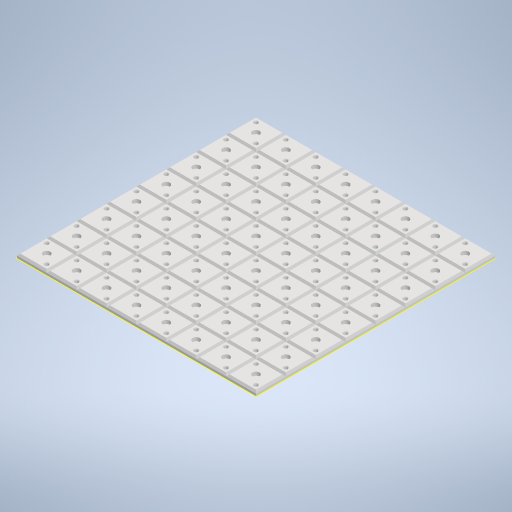
# Autodesk Inventor part: board-V2
Saved by Autodesk Inventor 2024.1 (Build 281209000, 209)
## iProperties
Created: 2025-07-31
Part Number: board-V2
Material: Generic
Document SubType Name: Modeling
Designer: iwheard
Density: 1 g/cm^3
Appearance: Default
Author: iwheard
Autodesk Inventor part; units mm, degrees
ref_plane "YZ Plane" through (0, 0, 0) normal (1, 0, 0) x (0, 1, 0)
ref_plane "XZ Plane" through (0, 0, 0) normal (0, 1, 0) x (-1, 0, 0)
ref_plane "XY Plane" through (0, 0, 0) normal (0, 0, 1) x (1, 0, 0)
sketch "Sketch1" plane through (0, 0, 0) normal (0, 1, 0) x (-1, 0, 0)
  line L0 (0, 0) -> (-25.5, 0)
  line L1 (-25.5, 0) -> (-25.5, -25.5)
  line L2 (-25.5, -25.5) -> (0, -25.5)
  line L3 (0, -25.5) -> (0, 0)
  dimension "d0" = 25.5
  dimension "d1" = 25.5
  constraints: 8 end point, 2 parallel, 1 horizontal, 1 perpendicular
  measures "d0" distance between parallel lines of L0 L2
  measures "d1" distance between parallel lines of L1 L3
extrude "Extrusion1" add sketch "Sketch1" along normal blind 3.5
chamfer "Chamfer1" distance 1.5 angle 45 4 edges at (12.75, 3.5, 0) (0, 3.5, -12.75) (25.5, 3.5, -12.75) (12.75, 3.5, -25.5)
sketch "Sketch2" plane through (0, 3.5, 0) normal (0, 1, 0) x (1, 0, 0)
  circle A0 centre (12.75, 12.75) radius 3
  line L0 (0, 0) -> (25.5, 0) projected
  line L1 (25.5, 25.5) -> (0, 25.5) projected
  line L2 (25.5, 0) -> (25.5, 25.5) projected
  line L3 (0, 25.5) -> (0, 0) projected
  dimension "d7" = 6
  dimension "d8" = 25.5
  dimension "d9" = 12.75
  dimension "d10" = 25.5
  dimension "d11" = 12.75
  constraints: 1 centre point
  measures "d7" diameter of A0
  measures "d8" distance between parallel lines of L0 L1
  measures "d9" distance from line of L1 A0.centre
  measures "d10" distance between parallel lines of L2 L3
  measures "d11" distance from line of L2 A0.centre
extrude "Extrusion2" cut sketch "Sketch2" against normal blind 3 contours A0
sketch "Sketch3" plane through (0, 3.5, 0) normal (0, 1, 0) x (1, 0, 0)
  circle A0 centre (20.5, 5) radius 1.5
  circle A1 centre (5, 20.5) radius 1.5
  line L0 (1.5, 24) -> (0, 25.5) projected
  line L1 (0, 25.5) -> (25.5, 0) construction
  line L2 (0, 0) -> (25.5, 0) projected
  dimension "d14" = 3
  dimension "d15" = 3
  dimension "d16" = 5
  dimension "d17" = 5
  constraints: 2 centre point, 2 end point, 2 point on line, 1 collinear
  measures "d14" diameter of A1
  measures "d15" diameter of A0
  measures "d16" horizontal distance of L0.end A1.centre
  measures "d17" distance from line of L2 A0.centre
extrude "Extrusion3" cut sketch "Sketch3" against normal blind 3
chamfer "Chamfer2" distance 0.5 angle 45 2 edges at (3.5, 3.5, -20.5) (19, 3.5, -5)
sketch "Sketch4" plane through (0, 0, 0) normal (0, -1, 0) x (1, 0, 0)
  line L0 (0, 0) -> (204, 0) projected
  line L1 (0, -204) -> (0, 0) projected
  line L2 (204, -204) -> (0, -204) projected
  line L3 (204, 0) -> (204, -204) projected
  line L4 (217, 13) -> (-13, 13)
  line L5 (-13, 13) -> (-13, -217)
  line L6 (-13, -217) -> (217, -217)
  line L7 (217, -217) -> (217, 13)
  dimension "d29" = 13
  constraints: 8 end point, 3 other
  measures "d29" distance between parallel lines of L4 L0
pattern_linear "Rectangular Pattern1" count 8 spacing 25.5 along (1, 0, 0) count 8 spacing 25.5 along (0, 0, -1)
sketch "Sketch5" plane through (0, 0, 0) normal (0, -1, 0) x (1, 0, 0)
  line L0 (0, 0) -> (204, 0) projected
  line L1 (0, -204) -> (0, 0) projected
  line L2 (204, -204) -> (0, -204) projected
  line L3 (204, 0) -> (204, -204) projected
equation "\"d9\" = 0.5 * d8"
equation "\"d11\" = 0.5 * d10"
body "Solid1"
